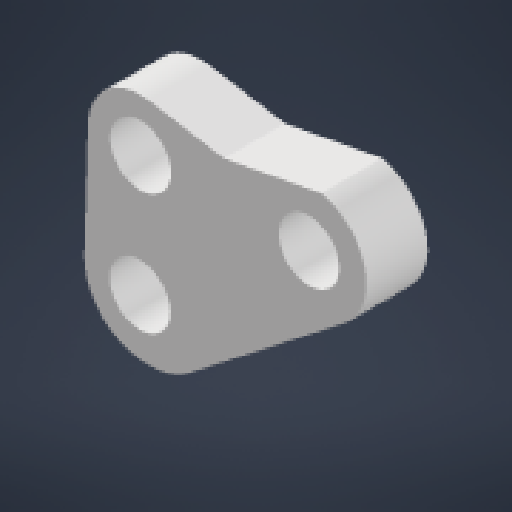
# Autodesk Inventor part: UpperLever
Saved by Autodesk Inventor 2024.1 (Build 281209000, 209)
## iProperties
Created: 2023-08-23
Part Number: UpperLever
Material: Generic
Document SubType Name: Modeling
Designer: Eleanor
Density: 1 g/cm^3
Appearance: Default
Author: Eleanor
Autodesk Inventor part; units mm, degrees
ref_plane "YZ Plane" through (0, 0, 0) normal (1, 0, 0) x (0, 1, 0)
ref_plane "XZ Plane" through (0, 0, 0) normal (0, 1, 0) x (-1, 0, 0)
ref_plane "XY Plane" through (0, 0, 0) normal (0, 0, 1) x (1, 0, 0)
sketch "Sketch1" plane through (0, 0, 0) normal (0, 0, 1) x (1, 0, 0)
  line L0 (6.8234, 3.035) -> (6.5538, -6.1146)
  line L1 (6.5538, -6.1146) -> (11.2152, -6.1146)
  line L2 (11.2152, -6.1146) -> (20.3343, 0.9713)
  circle A0 centre (18.3549, 3.2173) radius 2.9937
  circle A1 centre (18.3549, 3.2173) radius 1.5875
  line L3 (18.9975, 6.1413) -> (13.9136, 5.1722)
  circle A2 centre (9.5555, 3.1371) radius 2.734
  circle A3 centre (9.5555, 3.1371) radius 1.5875
  line L4 (13.9136, 5.1722) -> (10.0118, 5.8327)
  point P0 (0, 0)
  dimension "d0" = 3.175
  dimension "d1" = 3.175
  constraints: 10 end point, 4 centre point, 4 point on circle, 2 coincident, 1 horizontal, 1 tangent
  measures "d0" diameter of A1
  measures "d1" diameter of A3
extrude "Extrusion1" add sketch "Sketch1" along normal blind 3.175 contours A2 L4 L3 A0 L2 L1 L0 | A2 | A0 L3 L2
sketch "Sketch2" plane through (0, 0, 3.175) normal (0, 0, 1) x (1, 0, 0)
  circle A0 centre (9.525, -3.175) radius 1.5875
  point P0 (0, 0)
  constraints: 1 centre point
extrude "Extrusion2" cut sketch "Sketch2" against normal blind 3.175
fillet "Fillet1" radius 3.175 2 edges at (6.5538, -6.1146, 1.5875) (11.2152, -6.1146, 1.5875)
body "Solid1"
